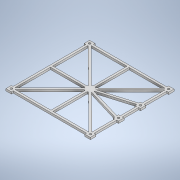
# Autodesk Inventor part: HexScrewGuide
Saved by Autodesk Inventor 2020 (Build 240168000, 168)
## iProperties
Created: 2023-12-26
Part Number: HexScrewGuide
Material: Generic
Document SubType Name: Modeling
Designer: smz3rm
Density: 1 g/cm^3
Appearance: Default
Author: smz3rm
Autodesk Inventor part; units mm, degrees
ref_plane "YZ Plane" through (0, 0, 0) normal (1, 0, 0) x (0, 1, 0)
ref_plane "XZ Plane" through (0, 0, 0) normal (0, 1, 0) x (-1, 0, 0)
ref_plane "XY Plane" through (0, 0, 0) normal (0, 0, 1) x (1, 0, 0)
sketch "Sketch1" plane through (0, 0, 0) normal (0, 1, 0) x (-1, 0, 0)
  line L0 (75, 65) -> (-75, 65)
  line L1 (-75, 65) -> (-75, -65)
  line L2 (-75, -65) -> (75, -65)
  line L3 (75, -65) -> (75, 65)
  line L4 (75, 65) -> (-75, -65) construction
  line L5 (-75, 65) -> (75, -65) construction
  line L6 (62.0096, 65) -> (62.0096, -65)
  line L7 (105, 0) -> (-105, 0) projected
  line L8 (0, -91) -> (0, 91) projected
  line L9 (-62.0096, 65) -> (-62.0096, -65)
  line L10 (61.6096, 65) -> (61.6096, -65)
  line L11 (-61.6096, 65) -> (-61.6096, -65)
  line L12 (-71, 61) -> (71, 61)
  line L13 (71, 61) -> (71, -61)
  line L14 (71, -61) -> (-71, -61)
  line L15 (-71, -61) -> (-71, 61)
  line L16 (61.6096, 61) -> (53.6096, 61)
  line L17 (53.6096, 61) -> (53.6096, 53)
  line L18 (53.6096, 53) -> (61.6096, 53)
  line L19 (61.6096, 53) -> (61.6096, 61)
  line L20 (61.6096, -61) -> (53.6096, -61)
  line L21 (53.6096, -61) -> (53.6096, -53)
  line L22 (53.6096, -53) -> (61.6096, -53)
  line L23 (-61.6096, 61) -> (-53.6096, 61)
  line L24 (-53.6096, 61) -> (-53.6096, 53)
  line L25 (-53.6096, 53) -> (-61.6096, 53)
  line L26 (-61.6096, 53) -> (-61.6096, 61)
  line L27 (-53.6096, -61) -> (-53.6096, -53)
  line L28 (-53.6096, -53) -> (-61.6096, -53)
  line L29 (-61.6096, -61) -> (-53.6096, -61)
  line L30 (-61.6096, 12) -> (-53.6096, 12)
  line L31 (-53.6096, 12) -> (-53.6096, 20)
  line L32 (-53.6096, 20) -> (-61.6096, 20)
  line L33 (-61.6096, 20) -> (-61.6096, 12)
  line L34 (-61.6096, -12) -> (-53.6096, -12)
  line L35 (-53.6096, -12) -> (-53.6096, -20)
  line L36 (-53.6096, -20) -> (-61.6096, -20)
  circle A0 centre (57.6096, 57) radius 1.55
  line L37 (61.6096, 57) -> (53.6096, 57)
  line L38 (57.6096, 61) -> (57.6096, 53)
  circle A1 centre (57.6096, -57) radius 1.55
  circle A2 centre (-57.6096, 57) radius 1.55
  circle A3 centre (-57.6096, -57) radius 1.55
  line L39 (-53.6096, 16) -> (-61.6096, 16)
  line L40 (-57.6096, 20) -> (-57.6096, 12)
  circle A4 centre (-57.6096, 16) radius 1.55
  circle A5 centre (-57.6096, -16) radius 1.55
  line L41 (53.6096, 57) -> (-53.6096, 57)
  line L42 (57.6096, 53) -> (57.6096, -53)
  line L43 (53.6096, -57) -> (-53.6096, -57)
  line L44 (-57.6096, -53) -> (-57.6096, -20)
  line L45 (-57.6096, -12) -> (-57.6096, 12)
  line L46 (-57.6096, 20) -> (-57.6096, 53)
  line L47 (53.6096, 53) -> (-53.6096, -53)
  line L48 (-53.6096, 53) -> (53.6096, -53)
  line L49 (0, 0) -> (57.6096, 0)
  line L50 (0, 0) -> (-57.6096, 0)
  line L51 (0, 0) -> (-53.6096, 16)
  line L52 (0, 0) -> (-53.6096, -16)
  circle A6 centre (0, 0) radius 6
  line L53 (53.6096, 55.1093) -> (3.0768, 5.1511)
  line L54 (53.6096, 58.5) -> (-53.6096, 58.5)
  line L55 (59.1096, 53) -> (59.1096, -53)
  line L56 (53.6096, -58.5) -> (-53.6096, -58.5)
  line L57 (-59.1096, -53) -> (-59.1096, -20)
  line L58 (-59.1096, -12) -> (-59.1096, 12)
  line L59 (-59.1096, 20) -> (-59.1096, 53)
  line L60 (-55.7432, 53) -> (-5.1859, 3.0177)
  line L61 (-5.9958, 0.2241) -> (-53.6096, 14.4346)
  line L62 (-53.6096, -17.5654) -> (-5.1378, -3.0988)
  line L63 (-3.0768, -5.1511) -> (-53.6096, -55.1093)
  line L64 (5.8095, -1.5) -> (57.6096, -1.5)
  line L65 (56.1096, 53) -> (56.1096, -53)
  line L66 (53.6096, 55.5) -> (-53.6096, 55.5)
  line L67 (55.7188, 52.9759) -> (5.1859, 3.0177)
  line L68 (5.8095, 1.5) -> (57.6096, 1.5)
  line L69 (-53.634, 55.1334) -> (-3.0768, 5.1511)
  line L70 (-5.1378, 3.0988) -> (-52.7517, 17.3093)
  line L71 (-5.1859, -3.0177) -> (-55.7188, -52.9759)
  line L72 (53.6096, -55.5) -> (-53.6096, -55.5)
  line L73 (-56.1096, -53) -> (-56.1096, -20)
  line L74 (-56.1096, -12) -> (-56.1096, 12)
  line L75 (-56.1096, 20) -> (-56.1096, 53)
  line L76 (-54.4676, -14.6907) -> (-5.9958, -0.2241)
  line L77 (3.0768, -5.1511) -> (53.6096, -55.1093)
  line L78 (5.1859, -3.0177) -> (55.7188, -52.9759)
  line L79 (1.5, 55.5) -> (1.5, 5.8095)
  line L80 (-1.5, 55.5) -> (-1.5, 5.8095)
  line L81 (1.5, -55.5) -> (1.5, -5.8095)
  line L82 (-1.5, -55.5) -> (-1.5, -5.8095)
  line L83 (-52.7517, 17.3093) -> (-53.6096, 17.5654)
  line L84 (55.7188, -52.9759) -> (55.7432, -53)
  line L85 (55.7188, 52.9759) -> (55.7432, 53)
  line L86 (-55.7188, -52.9759) -> (-55.7432, -53)
  point P0 (-61.6096, 61)
  point P1 (-61.6096, 0)
  point P2 (-71, 0)
  point P3 (4.2668, -4.2183)
  point P4 (56.1096, -1.5)
  point P5 (-4.2668, -4.2183)
  point P6 (-56.1096, -20)
  point P7 (1.5, -5.8095)
  point P8 (-1.5, -5.8095)
  point P9 (-1.5, 5.8095)
  point P10 (-3.0768, 5.1511)
  point P11 (-53.6096, 55.1093)
  point P12 (56.1096, 1.5)
  point P13 (4.2668, 4.2183)
  point P14 (-53.6096, -14.4346)
  point P15 (-5.7494, 1.7159)
  point P16 (-61.6096, -61)
  point P17 (61.6096, -61)
  point P18 (-5.3243, -3.1544)
  point P19 (5.1859, 3.0177)
  point P20 (-5.3243, 3.1544)
  dimension "d13" = 12
  dimension "d0" = 150
  dimension "d1" = 130
  dimension "d2" = 12.9904
  dimension "d3" = 0.4
  dimension "d4" = 4
  dimension "d5" = 8
  dimension "d6" = 8
  dimension "d7" = 8
  dimension "d8" = 8
  dimension "d9" = 12
  dimension "d10" = 3.1
  dimension "d11" = 3.1
  dimension "d14" = 3
  dimension "d15" = 3
  dimension "d16" = 3
  dimension "d17" = 3
  dimension "d18" = 3
  dimension "d19" = 3
  dimension "d20" = 3
  dimension "d21" = 3
  dimension "d22" = 3
  dimension "d23" = 3
  dimension "d24" = 3
  dimension "d25" = 3
  constraints: 170 end point, 55 symmetric about line, 31 point on line, 23 midpoint, 16 parallel, 10 perpendicular, 6 centre point, 5 collinear, 3 horizontal, 1 coincident, 1 vertical, 18 other
  measures "d0" distance of L2.end L1.end
  measures "d1" distance of L1.end L0.end
  measures "d2" distance between parallel lines of L3 L6
  measures "d3" distance between parallel lines of L6 L10
  measures "d4" distance between parallel lines of L0 L12
  measures "d5" distance of L18.end L17.end
  measures "d6" distance of L17.end L16.end
  measures "d7" distance of L32.end L31.end
  measures "d8" distance of L31.end L30.end
  measures "d9" distance between parallel lines of L7 L30
  measures "d10" diameter of A0
  measures "d11" diameter of A4
  measures "d14" distance between parallel lines of L65 L55
  measures "d15" distance between parallel lines of L67 L53
  measures "d16" distance between parallel lines of L66 L54
  measures "d17" distance between parallel lines of L64 L68
  measures "d18" distance between parallel lines of L56 L72
  measures "d19" distance between parallel lines of L63 L71
  measures "d20" distance between parallel lines of L62 L76
  measures "d21" distance between parallel lines of L61 L70
  measures "d22" distance between parallel lines of L60 L69
  measures "d23" distance between parallel lines of L74 L58
  measures "d24" distance between parallel lines of L77 L78
  measures "d25" distance between parallel lines of L80 L79
extrude "Extrusion1" add sketch "Sketch1" along normal blind 3 contours L10 L37 A0 L38 L12 | L10 L18 L38 A0 L37 | L38 A0 L37 L17 L12 | L12 L24 L25 L11 | L54 L17 L41 L8 | L8 L41 L24 L54 | L14 L21 L22 L10 | L55 L22 L42 L7 | L7 L42 L18 L55 | L41 L17 L66 L8 | L8 L66 L24 L41 | L38 L18 L17 L37 A0 | L42 L64 L65 L7 | L7 L65 L68 L42 | L32 L40 A4 L39 L11 | L25 L46 L32 L59 | L66 L79 A6 L8 | L8 A6 L80 L66 | L42 L68 L65 L18 | L56 L8 L43 L21 | L65 L64 A6 L7 | L7 A6 L68 L65 | L42 L22 L65 L64 | L11 L28 L27 L14 | L56 L27 L43 L8 | L39 A4 L40 L30 L11 | L25 L75 L32 L46 | A6 L47 L8 | L8 L48 A6 | L43 L8 L72 L21 | A6 L48 L7 | L7 L47 A6 | L43 L27 L72 L8 | L58 L30 L45 L7 | L7 L45 L34 L58 | L34 L35 L36 L11 | L32 L31 L39 A4 L40 | L52 A6 L7 | L48 A6 L8 | L8 A6 L47 | L51 A6 L48 | L7 A6 L51 | L47 A6 L52 | L17 L47 A6 L53 | L69 A6 L48 L24 | L85 L67 A6 L47 L18 | L22 L48 A6 L78 L84 | L57 L36 L44 L28 | L72 L82 A6 L8 | L8 A6 L81 L72 | L45 L30 L74 L7 | L7 L74 L34 L45 | A4 L39 L31 L30 L40 | L25 L48 A6 L70 L60 | A6 L63 L27 L47 | L47 L28 L86 L71 L62 A6 | L48 L21 L77 A6 | A6 L61 L31 L51 | L51 L31 L83 L70 L60 A6 | A6 L71 L62 L35 L52 | L52 L35 L76 A6 | L44 L36 L73 L28 | L70 A6 L60 | L62 L71 A6
equation "\"d0\" = BodyLength"
equation "\"d1\" = BodyWidth"
equation "\"d2\" = 0.433013 * BodyHeight"
equation "\"d4\" = SideThickness"
equation "\"d5\" = M3ScrewInsertBrim"
equation "\"d6\" = M3ScrewInsertBrim"
equation "\"d7\" = M3ScrewInsertBrim"
equation "\"d8\" = M3ScrewInsertBrim"
equation "\"d10\" = M3ScrewDia"
equation "\"d11\" = M3ScrewDia"
equation "\"BodyLength\" = 150"
equation "\"BodyWidth\" = 130"
equation "\"BodyHeight\" = 30"
equation "\"SideThickness\" = 4"
equation "\"M3ScrewInsertBrim\" = 8"
equation "\"M3ScrewDia\" = 3.1"
body "Solid1"
